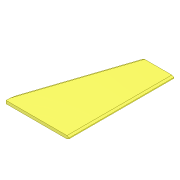
# Autodesk Inventor part: Foam_wing
Saved by Autodesk Inventor 2022 (Build 260153000, 153)
## iProperties
Created: 2022-06-29
Part Number: Foam_wing
Material: Generic
Document SubType Name: Modeling
Designer: dell
Density: 1 g/cm^3
Appearance: Smooth - Yellow
Author: dell
Autodesk Inventor part; units mm, degrees
ref_plane "YZ Plane" through (0, 0, 0) normal (1, 0, 0) x (0, 1, 0)
ref_plane "XZ Plane" through (0, 0, 0) normal (0, 1, 0) x (-1, 0, 0)
sketch "Sketch1" plane through (0, 0, 0) normal (0, 1, 0) x (-1, 0, 0)
  line L0 (0, 0) -> (600, 0)
  line L1 (600, 0) -> (600, -1000)
  line L2 (600, -1000) -> (0, -1000)
  line L3 (0, -1000) -> (0, 0)
  dimension "d0" = 1000
  dimension "d1" = 600
  constraints: 8 end point, 2 parallel, 1 horizontal, 1 perpendicular
  measures "d0" distance of L2.end L0.start
  measures "d1" distance of L0.start L0.end
extrude "Extrusion1" add sketch "Sketch1" along normal blind 28
sketch "Sketch2" plane through (0, 28, 0) normal (0, 1, 0) x (1, 0, 0)
  line L0 (-600, 1000) -> (-600, 0) projected
  line L1 (0, 1000) -> (-600, 1000) projected
  line L2 (0, 1000) -> (-600, 1000) projected
  line L3 (-600, 1000) -> (-600, 0) projected
  line L4 (-600, 0) -> (0, 0) projected
  line L5 (0, 0) -> (0, 1000) projected
  line L6 (-600, 100) -> (-300, 1000)
  dimension "d7" = 300
  dimension "d8" = 100
  constraints: 2 end point, 1 midpoint, 1 point on line
  measures "d7" distance of L1.start L6.end
  measures "d8" distance of L0.end L6.start
extrude "Extrusion2" cut sketch "Sketch2" against normal blind 200 contours L1 L6 L0
ref_plane "Work Plane1" through (0, 14, 0) normal (0, 1, 0) x (1, 0, 0)
sketch "Sketch3" plane through (0, 28, 0) normal (0, 1, 0) x (1, 0, 0)
  circle A0 centre (-305, 20) radius 8
  line L0 (0, 0) -> (0, 1000) projected
  line L1 (-600, 0) -> (0, 0) projected
  circle A1 centre (-395, 20) radius 8
  circle A2 centre (-350, 75) radius 8
  circle A3 centre (-350, 160) radius 8
  dimension "d9" = 16
  dimension "d10" = 305
  dimension "d11" = 20
  dimension "d12" = 16
  dimension "d13" = 395
  dimension "d14" = 20
  dimension "d15" = 16
  dimension "d16" = 350
  dimension "d17" = 75
  dimension "d18" = 16
  dimension "d19" = 350
  dimension "d20" = 160
  constraints: 4 centre point
  measures "d9" diameter of A0
  measures "d10" distance from line of L0 A0.centre
  measures "d11" distance from line of L1 A0.centre
  measures "d12" diameter of A1
  measures "d13" distance from line of L0 A1.centre
  measures "d14" distance from line of L1 A1.centre
  measures "d15" diameter of A2
  measures "d16" distance from line of L0 A2.centre
  measures "d17" distance from line of L1 A2.centre
  measures "d18" diameter of A3
  measures "d19" distance from line of L0 A3.centre
  measures "d20" distance from line of L1 A3.centre
extrude "Extrusion3" [suppressed]
chamfer "Chamfer1" distance 20 distance2 10 1 edges at (0, 28, -500) measured on face at (-300, 28, -366.6667)
chamfer "Chamfer2" distance 10 distance2 20 1 edges at (0, 0, -500) measured on face at (0, 6, -333.3333)
chamfer "Chamfer3" distance 20 distance2 10 1 edges at (-450, 28, -550) measured on face at (-306.6667, 28, -366.6667)
chamfer "Chamfer4" distance 20 distance2 10 1 edges at (-450, 0, -550) measured on face at (-306.6667, 0, -366.6667)
body "Solid1"
